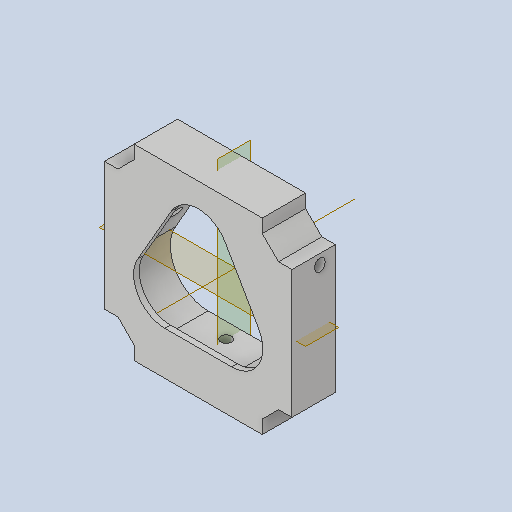
# Autodesk Inventor part: 20_Cube_Insert_Filter_25mm
Saved by Autodesk Inventor 2023 (Build 270158000, 158)
## iProperties
Created: 2019-07-01
Part Number: 20_Cube_Insert_Filter_25mm
Material: Generic
Document SubType Name: Modeling
Designer: diederichbenedict
Density: 1 g/cm^3
Appearance: Default
Author: diederichbenedict
Autodesk Inventor part; units mm, degrees
ref_plane "YZ Plane" through (0, 0, 0) normal (1, 0, 0) x (0, 1, 0)
ref_plane "XZ Plane" through (0, 0, 0) normal (0, 1, 0) x (-1, 0, 0)
ref_plane "Work Plane1" through (-56.3599, 0, 22) normal (0, 0, -1) x (-1, 0, 0)
sketch "Sketch1" plane through (-56.3599, 0, 22) normal (0, 0, -1) x (-1, 0, 0)
  line L0 (-4.0299, -0.3538) -> (-2.2322, 1.4439) construction
  arc A0 (-1.4439, 2.2322) -> (-2.2322, 1.4439) centre (-0.9299, 0.9299) ccw construction
  line L1 (-1.4439, 2.2322) -> (0.3538, 4.0299) construction
  line L2 (-37.8299, 42.8299) -> (-37.8299, 37.8299) construction
  line L3 (-37.8299, 37.8299) -> (-42.9208, 37.8299) construction
  line L4 (-37.8299, 42.2137) -> (-37.8299, 45.8299) construction
  line L5 (-37.8299, 45.8299) -> (-4.0299, 45.8299) construction
  line L6 (-4.0299, 45.8299) -> (-4.0299, 42.2137) construction
  line L7 (-4.0299, 4.0299) -> (0.3538, 4.0299) projected
  circle A1 centre (-20.9299, 20.9299) radius 17.5 projected
  line L8 (-20.9299, 58.9723) -> (17.1124, 20.9299) construction
  line L9 (17.1124, 20.9299) -> (-20.9299, -17.1124) construction
  line L10 (-20.9299, -17.1124) -> (-58.9723, 20.9299) construction
  line L11 (-58.9723, 20.9299) -> (-20.9299, 58.9723) construction
  line L12 (-20.9299, 58.9723) -> (-20.9299, -17.1124) construction
  line L13 (17.1124, 20.9299) -> (-58.9723, 20.9299) construction
  line L14 (-20.9299, 58.9723) -> (32.8701, 58.9723) construction
  line L15 (-43.4299, 43.4299) -> (1.5701, 43.4299) construction
  line L16 (1.5701, 43.4299) -> (1.5701, -1.5701) construction
  line L17 (1.5701, -1.5701) -> (-43.4299, -1.5701) construction
  line L18 (-43.4299, -1.5701) -> (-43.4299, 43.4299) construction
  line L19 (-43.4299, 43.4299) -> (1.5701, -1.5701) construction
  line L20 (1.5701, 43.4299) -> (-43.4299, -1.5701) construction
  line L21 (-43.4299, 5.3876) -> (-43.4299, 36.4723)
  line L22 (-43.4299, 36.4723) -> (-36.4723, 43.4299)
  line L23 (-36.4723, 43.4299) -> (-5.3876, 43.4299)
  line L24 (-5.3876, 43.4299) -> (1.5701, 36.4723)
  line L25 (1.5701, 36.4723) -> (1.5701, 5.3876)
  line L26 (1.5701, 5.3876) -> (-5.3876, -1.5701)
  line L27 (-5.3876, -1.5701) -> (-36.4723, -1.5701)
  line L28 (-36.4723, -1.5701) -> (-43.4299, 5.3876)
  line L29 (-4.0299, 42.2137) -> (-37.8299, 42.2137) projected
  line L30 (-4.0299, -0.3538) -> (-4.0299, 4.0299) projected
  circle A2 centre (-20.9299, 20.9299) radius 1.5
  line L31 (-10.9299, 10.9299) -> (-30.9299, 10.9299) construction
  line L32 (-30.9299, 10.9299) -> (-30.9299, 30.9299) construction
  line L33 (-30.9299, 30.9299) -> (-10.9299, 30.9299) construction
  line L34 (-10.9299, 30.9299) -> (-10.9299, 10.9299) construction
  line L35 (-10.9299, 10.9299) -> (-30.9299, 30.9299) construction
  line L36 (-30.9299, 10.9299) -> (-10.9299, 30.9299) construction
  circle A3 centre (-30.9299, 30.9299) radius 1.4
  circle A4 centre (-30.9299, 10.9299) radius 1.4
  circle A5 centre (-10.9299, 10.9299) radius 1.4
  line L37 (-45.8299, 37.8299) -> (-42.0723, 37.8299) construction
  line L38 (-42.1723, 37.7299) -> (-45.8299, 37.7299)
  line L39 (-45.8299, 37.7299) -> (-45.8299, 4.1299)
  line L40 (-45.8299, 4.1299) -> (-42.1723, 4.1299)
  line L41 (-42.1723, 4.1299) -> (-42.1723, 37.7299)
  line L42 (-45.8299, 4.0299) -> (-42.0723, 4.0299) construction
  line L43 (-45.8299, 37.8299) -> (-42.0723, 37.8299) projected
  line L44 (-37.7299, 45.8299) -> (-4.1299, 45.8299)
  line L45 (-4.1299, 45.8299) -> (-4.1299, 42.1723)
  line L46 (-4.1299, 42.1723) -> (-37.7299, 42.1723)
  line L47 (-37.7299, 42.1723) -> (-37.7299, 45.8299)
  line L48 (0.4701, 37.8299) -> (0.4701, 4.0299) construction
  line L49 (0.4701, 4.0299) -> (3.9701, 4.0299) construction
  line L50 (3.9701, 37.8299) -> (3.9701, 4.0299) construction
  line L51 (0.4701, 37.8299) -> (3.9701, 37.8299) construction
  line L52 (-45.8299, -3.9701) -> (-4.0299, -3.9701) construction
  line L53 (0.3124, 37.7299) -> (3.9701, 37.7299)
  line L54 (3.9701, 37.7299) -> (3.9701, 4.1299)
  line L55 (3.9701, 4.1299) -> (0.3124, 4.1299)
  line L56 (0.3124, 4.1299) -> (0.3124, 37.7299)
  line L57 (-4.1713, -0.3538) -> (-37.7299, -0.3538)
  line L58 (-37.7299, -0.3538) -> (-37.7299, -3.9701)
  line L59 (-37.7299, -3.9701) -> (-4.1713, -3.9701)
  line L60 (-4.1713, -3.9701) -> (-4.1713, -0.3538)
  point P0 (-37.8299, 4.0299)
  dimension "d18" = 53.8
  dimension "d19" = 45
  dimension "d20" = 53.8
  dimension "d21" = 45
  dimension "d22" = 45
  dimension "d30" = 20
  dimension "d31" = 20
  dimension "d32" = 2.8
  dimension "d33" = 2.8
  dimension "d34" = 2.8
  dimension "d35" = 3
  dimension "d36" = 0.1
  dimension "d37" = 0.1
  dimension "d38" = 0.1
  dimension "d39" = 0.1
  constraints: 86 end point, 21 point on line, 14 parallel, 8 perpendicular, 7 horizontal, 7 midpoint, 4 centre point, 4 coincident, 1 equal length
  measures "d18" distance of L8.start L8.end
  measures "d19" angle of L8 L14
  measures "d20" distance of L8.end L9.end
  measures "d21" distance of L16.end L17.end
  measures "d22" distance of L15.end L16.end
  measures "d30" distance of L32.end L33.end
  measures "d31" distance of L31.end L32.end
  measures "d32" diameter of A3
  measures "d33" diameter of A4
  measures "d34" diameter of A5
  measures "d35" diameter of A2
  measures "d36" distance between parallel lines of L38 L43
  measures "d37" distance between parallel lines of L40 L42
  measures "d38" distance between parallel lines of L45 L6
  measures "d39" distance between parallel lines of L4 L47
extrude "Extrusion1" add sketch "Sketch1" along normal blind 10 contours L30 L26 L57 L28 L41 L22 L46 L24 L56 L7 | L7 L26 L30 | L56 L24 L25 L26 | L26 L25 L24 L53 L54 L55 | L60 L59 L58 L57 L28 L27 L26 | L26 L27 L28 L57 | L46 L22 L29 L24 | L24 L29 L45 | L40 L39 L38 L22 L21 L28 | L28 L21 L22 L41 | L29 L22 L23 L24 | L24 L23 L22 L29 L47 L44 L45 | L47 L29 L22 | A1 | A2 | A3 | A4 | A5
sketch "Skizze4" plane through (-56.3599, 0, 12) normal (0, 0, -1) x (-1, 0, 0)
  line L0 (-37.7299, 42.1723) -> (-42.1723, 37.7299) projected
  line L1 (-42.1723, 37.7299) -> (-45.8299, 37.7299) projected
  line L2 (-45.8299, 37.7299) -> (-45.8299, 4.1299) construction
  line L3 (-45.8299, 4.1299) -> (-42.1723, 4.1299) projected
  line L4 (-42.1723, 4.1299) -> (-37.6885, -0.3538) projected
  line L5 (-37.6885, -0.3538) -> (-37.7299, -0.3538) projected
  line L6 (-37.7299, -0.3538) -> (-37.7299, -3.9701) projected
  line L7 (-37.7299, -3.9701) -> (-4.1713, -3.9701) construction
  line L8 (-4.1713, -3.9701) -> (-4.1713, -0.3538) projected
  line L9 (-4.1713, -0.3538) -> (0.3124, 4.1299) projected
  line L10 (0.3124, 4.1299) -> (3.9701, 4.1299) projected
  line L11 (3.9701, 4.1299) -> (3.9701, 37.7299) construction
  line L12 (3.9701, 37.7299) -> (0.3124, 37.7299) projected
  line L13 (0.3124, 37.7299) -> (-4.1299, 42.1723) projected
  line L14 (-4.1299, 42.1723) -> (-4.1299, 45.8299) projected
  line L15 (-4.1299, 45.8299) -> (-37.7299, 45.8299) construction
  line L16 (-37.7299, 45.8299) -> (-37.7299, 42.1723) projected
  line L17 (-37.9299, 46.0299) -> (-3.9299, 46.0299) construction
  line L18 (-3.9299, 46.0299) -> (-3.9299, 42.2551)
  line L19 (-3.9299, 42.2551) -> (0.3953, 37.9299)
  line L20 (0.3953, 37.9299) -> (4.1701, 37.9299)
  line L21 (4.1701, 37.9299) -> (4.1701, 3.9299) construction
  line L22 (4.1701, 3.9299) -> (0.3953, 3.9299)
  line L23 (0.3953, 3.9299) -> (-3.9713, -0.4367)
  line L24 (-3.9713, -0.4367) -> (-3.9713, -4.1701)
  line L25 (-3.9713, -4.1701) -> (-37.9299, -4.1701) construction
  line L26 (-37.9299, -4.1701) -> (-37.9299, -0.3953)
  line L27 (-37.9299, -0.3953) -> (-42.2551, 3.9299)
  line L28 (-42.2551, 3.9299) -> (-46.0299, 3.9299)
  line L29 (-46.0299, 3.9299) -> (-46.0299, 37.9299) construction
  line L30 (-46.0299, 37.9299) -> (-42.2551, 37.9299)
  line L31 (-42.2551, 37.9299) -> (-37.9299, 42.2551)
  line L32 (-37.9299, 42.2551) -> (-37.9299, 46.0299)
  line L33 (-45.8299, 37.7299) -> (-45.8299, 37.9299)
  line L34 (-4.1299, 45.8299) -> (-37.7299, 45.8299) projected
  line L35 (-37.7299, 45.8299) -> (-37.9299, 45.8299)
  line L36 (-4.1299, 45.8299) -> (-3.9299, 45.8299)
  line L37 (3.9701, 37.7299) -> (3.9701, 37.9299)
  line L38 (3.9701, 4.1299) -> (3.9701, 37.7299) projected
  line L39 (3.9701, 4.1299) -> (3.9701, 3.9299)
  line L40 (-4.1713, -3.9701) -> (-3.9713, -3.9701)
  line L41 (-37.7299, -3.9701) -> (-37.9299, -3.9701)
  line L42 (-45.8299, 4.1299) -> (-45.8299, 3.9299)
  point P0 (-56.3599, 0)
  dimension "d40" = 0.2
  constraints: 48 end point, 12 point on line, 4 perpendicular, 15 other
  measures "d40" distance between parallel lines of L15 L17
extrude "IM_offset" add sketch "Skizze4" against normal up to surface (10 mm away)
ref_plane "Arbeitsebene5" through (-35.4299, 3.9299, 22) normal (-1, 0, 0) x (0, 0, 1)
ref_plane "Arbeitsebene6" through (-18.4299, 20.9299, 22) normal (0, 1, 0) x (-1, 0, 0)
sketch "Sketch33" plane through (-56.3599, 0, 12) normal (0, 0, -1) x (-1, 0, 0)
  circle A0 centre (-20.9299, 20.9299) radius 15.24 construction
  circle A1 centre (-20.9299, 20.9299) radius 15.14 construction
  line L0 (-12.0272, 5.7899) -> (-29.8327, 5.7899)
  line L1 (-38.4929, 20.7899) -> (-29.5902, 36.2099)
  line L2 (-12.2697, 36.2099) -> (-3.3669, 20.7899)
  line L3 (-42.2551, 3.9299) -> (-45.8299, 3.9299) projected
  arc A2 (-12.0272, 5.7899) -> (-3.3669, 20.7899) centre (-12.0272, 15.7899) ccw
  arc A3 (-38.4929, 20.7899) -> (-29.8327, 5.7899) centre (-29.8327, 15.7899) ccw
  arc A4 (-12.2697, 36.2099) -> (-29.5902, 36.2099) centre (-20.9299, 31.2099) ccw
  point P0 (-56.3599, 0)
  point P1 (5.2933, 5.7899)
  point P2 (-47.1532, 5.7899)
  point P3 (-20.9299, 51.2099)
  dimension "d184" = 0.1
  dimension "d185" = 0
  dimension "d186" = 10
  constraints: 7 tangent, 6 end point, 6 point on circle, 6 point on line, 4 centre point, 2 equal radius, 1 coincident, 7 other
  measures "d184" radial gap between concentric circles of A0 A1
  measures "d185" angle of L0 L3
  measures "d186" radius of A2
extrude "Extrusion27" cut sketch "Sketch33" against normal blind 10
sketch "Sketch34" plane through (-56.3599, 0, 22) normal (0, 0, 1) x (1, 0, 0)
  arc A0 (29.8327, 5.7899) -> (38.4929, 20.7899) centre (29.8327, 15.7899) ccw projected
  line L0 (29.8327, 5.7899) -> (12.0272, 5.7899) projected
  arc A1 (3.3669, 20.7899) -> (12.0272, 5.7899) centre (12.0272, 15.7899) ccw projected
  line L1 (3.3669, 20.7899) -> (12.2697, 36.2099) projected
  arc A2 (29.5902, 36.2099) -> (12.2697, 36.2099) centre (20.9299, 31.2099) ccw projected
  line L2 (29.5902, 36.2099) -> (38.4929, 20.7899) projected
  line L3 (3.9713, -3.9701) -> (37.9299, -3.9701) projected
  line L4 (37.9299, -3.9701) -> (37.9299, -0.3953) projected
  line L5 (37.9299, -0.3953) -> (42.2551, 3.9299) projected
  line L6 (42.2551, 3.9299) -> (45.8299, 3.9299) projected
  line L7 (45.8299, 3.9299) -> (45.8299, 37.9299) projected
  line L8 (45.8299, 37.9299) -> (42.2551, 37.9299) projected
  line L9 (42.2551, 37.9299) -> (37.9299, 42.2551) projected
  line L10 (37.9299, 42.2551) -> (37.9299, 45.8299) projected
  line L11 (37.9299, 45.8299) -> (3.9299, 45.8299) projected
  line L12 (3.9299, 45.8299) -> (3.9299, 42.2551) projected
  line L13 (3.9299, 42.2551) -> (-0.3953, 37.9299) projected
  line L14 (-0.3953, 37.9299) -> (-3.9701, 37.9299) projected
  line L15 (-3.9701, 37.9299) -> (-3.9701, 3.9299) projected
  line L16 (-3.9701, 3.9299) -> (-0.3953, 3.9299) projected
  line L17 (-0.3953, 3.9299) -> (3.9713, -0.4367) projected
  line L18 (3.9713, -0.4367) -> (3.9713, -3.9701) projected
  circle A3 centre (20.9299, 20.9299) radius 13.5001 construction
  circle A4 centre (20.9299, 20.9299) radius 13.4001
  line L19 (12.0272, 7.5298) -> (29.8327, 7.5298)
  arc A5 (29.8327, 7.5298) -> (36.9861, 19.92) centre (29.8327, 15.7899) ccw
  line L20 (36.9861, 19.92) -> (28.0834, 35.34)
  arc A6 (28.0834, 35.34) -> (13.7765, 35.34) centre (20.9299, 31.2099) ccw
  line L21 (13.7765, 35.34) -> (4.8737, 19.92)
  arc A7 (4.8737, 19.92) -> (12.0272, 7.5298) centre (12.0272, 15.7899) ccw
  point P0 (56.3599, 0)
  dimension "d189" = 0.1
  constraints: 6 end point, 6 point on circle, 4 centre point, 1 tangent, 5 other
  measures "d189" radial gap between concentric circles of A3 A4
extrude "Extrusion28" add sketch "Sketch34" along normal blind 1.5 contours L0 A1 L1 A2 L2 A0 | L18 L17 L16 L15 L14 L13 L12 L11 L10 L9 L8 L7 L6 L5 L4 L3
sketch "Sketch35" plane through (-52.3885, -3.9701, 12) normal (0, -1, 0) x (1, 0, 0)
  line L0 (0, 0) -> (0, 11.5) projected
  line L1 (0, 0) -> (33.9586, 0) projected
  line L2 (33.9586, 0) -> (33.9586, 11.5) projected
  line L3 (0, 11.5) -> (33.9586, 11.5) projected
  circle A0 centre (16.9586, 4.104) radius 1.4
  point P0 (52.3885, -12)
  dimension "d192" = 2.8
  constraints: 1 centre point
  measures "d192" diameter of A0
extrude "Extrusion29" cut sketch "Sketch35" along normal mid plane 30 contours A0
pattern_circular "Circular Pattern2" count 3 over 360 about axis through (-35.4299, 20.9299, 22) along (0, 0, 1) of "Extrusion29"
body "Solid1"
